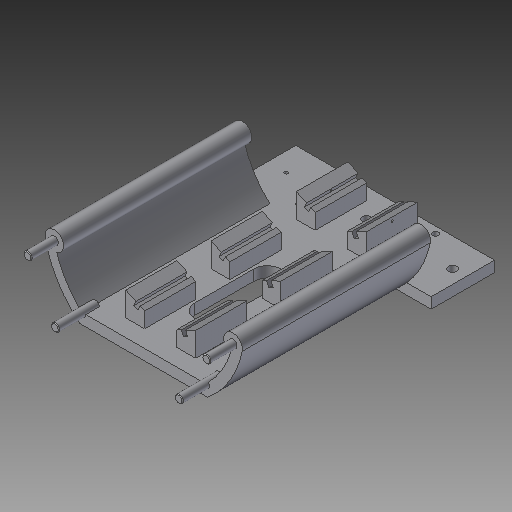
# Autodesk Inventor part: 3214_Bed Rail End_V1
Saved by Autodesk Inventor 2020 (Build 240168000, 168)
## iProperties
Created: 2019-06-18
Part Number: 3214_Bed Rail End_V1
Material: Acetal Resin, White
Document SubType Name: Sheet Metal
Designer: MPI
Density: 1.425 g/cm^3
Sheet Metal Rule: Default_mm
Appearance: Smooth - White
Mass: 455.781 g
Surface Area: 903.238 cm^2
Volume: 319.846 cm^3
Author: MPI
Autodesk Inventor part; units mm, degrees
ref_plane "YZ Plane" through (0, 0, 0) normal (1, 0, 0) x (0, 1, 0)
sketch "Sketch19" plane through (0, 0, 0) normal (0, 0, 1) x (1, 0, 0)
  line L0 (47.55, -58) -> (-47.55, -58)
  line L1 (-100, -14) -> (156, -14) construction
  arc A0 (47.55, -58) -> (73.6817, -14) centre (0, 0) ccw
  arc A1 (-73.6817, -14) -> (-47.55, -58) centre (0, 0) ccw
  arc A2 (-64.7514, -20.7668) -> (-73.3933, -15.4412) centre (-66.5432, -14) ccw
  arc A3 (73.3933, -15.4412) -> (64.7514, -20.7668) centre (66.5432, -14) ccw
  arc A4 (-67.6299, -7.0849) -> (-64.8992, -20.3) centre (0, 0) ccw construction
  arc A5 (-64.7514, -20.7668) -> (-46.0869, -50) centre (0, 0) ccw
  arc A6 (46.0869, -50) -> (64.7514, -20.7668) centre (0, 0) ccw
  arc A7 (64.8058, -20.5962) -> (67.6299, -7.0849) centre (0, 0) ccw construction
  line L2 (0, 0) -> (-33.9351, 15.8242) construction
  line L3 (0, 0) -> (37.291, 17.3891) construction
  line L4 (0, 0) -> (0, -41) construction
  line L5 (0, 0) -> (-21.2237, -45.5143) construction
  line L6 (0, 0) -> (17.7082, -37.9755) construction
  line L7 (-12, -38.5394) -> (-12, -50)
  line L8 (12, -38.5394) -> (12, -50)
  line L9 (-26, -32.0111) -> (-26, -50)
  line L10 (26, -32.0111) -> (26, -50)
  line L11 (-18.4455, -35.5339) -> (-20.1359, -39.1591)
  line L12 (-20.1359, -39.1591) -> (-17.0545, -40.596)
  line L13 (-17.0545, -40.596) -> (-15.364, -36.9708)
  line L14 (15.364, -36.9708) -> (17.0545, -40.596)
  line L15 (17.0545, -40.596) -> (20.1359, -39.1591)
  line L16 (20.1359, -39.1591) -> (18.4455, -35.5339)
  line L17 (-12, -38.5394) -> (-15.364, -36.9708)
  line L18 (-18.4455, -35.5339) -> (-26, -32.0111)
  line L19 (12, -38.5394) -> (15.364, -36.9708)
  line L20 (18.4455, -35.5339) -> (26, -32.0111)
  line L21 (-46.0869, -50) -> (-26, -50)
  line L22 (-12, -50) -> (12, -50)
  line L23 (26, -50) -> (46.0869, -50)
  dimension "d378" = 58
  dimension "d379" = 14
  dimension "d381" = 75
  dimension "d383" = 75
  dimension "d384" = 14
  dimension "d385" = 14
  dimension "d389" = 25
  dimension "d390" = 25
  dimension "d391" = 90
  dimension "d392" = 90
  dimension "d393" = 24
  dimension "d394" = 12
  dimension "d395" = 14
  dimension "d396" = 14
  dimension "d399" = 3.4
  dimension "d400" = 4
  dimension "d401" = 1.7
  dimension "d402" = 3.4
  dimension "d403" = 1.7
  dimension "d404" = 4
  constraints: 48 end point, 20 point on circle, 11 perpendicular, 8 centre point, 8 parallel, 4 horizontal, 2 coincident, 2 point on line, 2 vertical
  measures "d378" distance from line of L0 point (0, 0)
  measures "d379" distance from line of L1 point (0, 0)
  measures "d381" radius of A1
  measures "d383" radius of A0
  measures "d384" diameter of A2
  measures "d385" diameter of A3
  measures "d389" angle of L4 L6
  measures "d390" angle of L4 L5
  measures "d391" angle of L5 L2
  measures "d392" angle of L6 L3
  measures "d393" distance between parallel lines of L8 L7
  measures "d394" distance between parallel lines of L4 L7
  measures "d395" distance between parallel lines of L7 L9
  measures "d396" distance between parallel lines of L10 L8
  measures "d399" distance between parallel lines of L13 L11
  measures "d400" distance of L12.end L13.end
  measures "d401" distance between parallel lines of L5 L13
  measures "d402" distance between parallel lines of L16 L14
  measures "d403" distance between parallel lines of L6 L14
  measures "d404" distance of L14.start L14.end
extrude "Extrusion17" add sketch "Sketch19" along normal blind 140
sketch "Sketch20" plane through (0, 0, 0) normal (0, 0, -1) x (-1, 0, 0)
  line L0 (74, -50) -> (74, -58)
  line L1 (74, -58) -> (-74, -58)
  line L2 (-74, -58) -> (-74, -50)
  line L3 (47.55, -58) -> (-47.55, -58) projected
  line L4 (26, -50) -> (46.0869, -50) projected
  line L5 (-46.0869, -50) -> (-26, -50) projected
  line L6 (-26, -50) -> (-26, -32.0111)
  line L7 (-26, -32.0111) -> (-18.4455, -35.5339)
  line L8 (-18.4455, -35.5339) -> (-20.1359, -39.1591)
  line L9 (-20.1359, -39.1591) -> (-17.0545, -40.596)
  line L10 (-17.0545, -40.596) -> (-15.364, -36.9708)
  line L11 (-15.364, -36.9708) -> (-12, -38.5394)
  line L12 (-12, -38.5394) -> (-12, -50)
  line L13 (-12, -50) -> (12, -50) projected
  line L14 (12, -50) -> (12, -38.5394)
  line L15 (12, -38.5394) -> (15.364, -36.9708)
  line L16 (17.0545, -40.596) -> (20.1359, -39.1591)
  line L17 (20.1359, -39.1591) -> (18.4455, -35.5339)
  line L18 (18.4455, -35.5339) -> (26, -32.0111)
  line L19 (26, -32.0111) -> (26, -50)
  line L20 (26, -32.0111) -> (26, -50) projected
  line L21 (20.1359, -39.1591) -> (18.4455, -35.5339) projected
  line L22 (12, -50) -> (12, -38.5394) projected
  line L23 (12, -38.5394) -> (15.364, -36.9708) projected
  line L24 (15.364, -36.9708) -> (17.0545, -40.596)
  line L25 (15.364, -36.9708) -> (17.0545, -40.596) projected
  line L26 (-26, -50) -> (-26, -32.0111) projected
  line L27 (-12, -38.5394) -> (-12, -50) projected
  line L28 (-20.1359, -39.1591) -> (-17.0545, -40.596) projected
  line L29 (-17.0545, -40.596) -> (-15.364, -36.9708) projected
  line L30 (-15.364, -36.9708) -> (-12, -38.5394) projected
  line L31 (-26, -32.0111) -> (-18.4455, -35.5339) projected
  line L32 (-18.4455, -35.5339) -> (-20.1359, -39.1591) projected
  line L33 (-74, -50) -> (-26, -50)
  line L34 (-12, -50) -> (12, -50)
  line L35 (26, -50) -> (74, -50)
  point P0 (0, 0)
  dimension "d407" = 148
  dimension "d408" = 74
  constraints: 44 end point, 16 collinear, 8 perpendicular, 5 parallel, 3 horizontal, 3 point on line, 2 vertical
  measures "d407" distance between parallel lines of L0 L2
  measures "d408" distance from line of point (0, 0) L2
extrude "Extrusion18" add sketch "Sketch20" along normal blind 38.1
sketch "Sketch21" plane through (-12, -50, 140) normal (0, 1, 0) x (1, 0, 0)
  line L0 (48, 0) -> (-24, 0)
  line L1 (-24, 0) -> (-24, 12.7)
  line L2 (-24, 12.7) -> (48, 12.7)
  line L3 (48, 12.7) -> (48, 0)
  line L4 (48, 50.8) -> (-24, 50.8)
  line L5 (-24, 50.8) -> (-24, 76.2)
  line L6 (-24, 76.2) -> (48, 76.2)
  line L7 (48, 76.2) -> (48, 50.8)
  line L8 (48, 114.3) -> (-24, 114.3)
  line L9 (-24, 114.3) -> (-24, 139.7)
  line L10 (-24, 139.7) -> (48, 139.7)
  line L11 (48, 139.7) -> (48, 114.3)
  line L12 (24, 0) -> (0, 0) projected
  line L13 (38, 178.1) -> (38, 0) projected
  line L14 (-14, 178.1) -> (-14, 0) projected
  point P0 (12, 140)
  dimension "d412" = 10
  dimension "d413" = 10
  dimension "d414" = 12.7
  dimension "d415" = 38.1
  dimension "d416" = 25.4
  dimension "d417" = 38.1
  dimension "d418" = 25.4
  constraints: 24 end point, 6 parallel, 3 horizontal, 3 perpendicular, 3 point on line, 2 collinear
  measures "d412" distance between parallel lines of L13 L3
  measures "d413" distance between parallel lines of L14 L1
  measures "d414" distance of L0.end L1.end
  measures "d415" distance between parallel lines of L4 L2
  measures "d416" distance between parallel lines of L6 L4
  measures "d417" distance between parallel lines of L8 L6
  measures "d418" distance between parallel lines of L8 L10
extrude "Extrusion19" cut sketch "Sketch21" along normal up to next contours L0 L13 L2 L3 | L0 L14 L2 L13 | L14 L0 L1 L2 | L13 L6 L7 L4 | L4 L14 L6 L13 | L4 L5 L6 L14 | L13 L10 L11 L8 | L8 L14 L10 L13 | L8 L9 L10 L14
sketch "Sketch22" plane through (0, 0, 140) normal (0, 0, 1) x (1, 0, 0)
  arc A0 (-64.7514, -20.7668) -> (-73.3933, -15.4412) centre (-66.5432, -14) ccw projected
  circle A1 centre (-66.5432, -14) radius 3
  arc A2 (73.3933, -15.4412) -> (64.7514, -20.7668) centre (66.5432, -14) ccw projected
  circle A3 centre (66.5432, -14) radius 3
  arc A4 (-64.7514, -20.7668) -> (-46.0869, -50) centre (0, 0) ccw projected
  circle A5 centre (-46.0869, -50) radius 3
  arc A6 (46.0869, -50) -> (64.7514, -20.7668) centre (0, 0) ccw projected
  circle A7 centre (46.0869, -50) radius 3
  dimension "d421" = 6
  dimension "d422" = 6
  dimension "d423" = 6
  dimension "d424" = 6
  constraints: 4 centre point, 2 coincident, 2 other
  measures "d421" diameter of A1
  measures "d422" diameter of A3
  measures "d423" diameter of A5
  measures "d424" diameter of A7
extrude "Extrusion20" add sketch "Sketch22" along normal blind 20 and the other way blind 10
fillet "Fillet1" radius 0.5 4 edges at (-69.5432, -14, 160) (-49.0869, -50, 160) (43.0869, -50, 160) (63.5432, -14, 160)
sketch "Sketch23" plane through (55.9017, -50, 0) normal (0, 1, 0) x (1, 0, 0)
  circle A0 centre (-115.9017, 26.1) radius 1.3
  line L0 (-129.9017, 0) -> (-129.9017, 38.1) projected
  line L1 (18.0983, 0) -> (18.0983, 38.1) projected
  line L2 (-129.9017, 38.1) -> (-81.9017, 38.1) projected
  line L3 (-29.9017, 38.1) -> (18.0983, 38.1) projected
  circle A1 centre (-55.9017, 26.1) radius 3.25
  line L4 (-67.9017, 38.1) -> (-43.9017, 38.1) projected
  circle A2 centre (8.0983, 26.1) radius 3.25
  point P0 (-55.9017, 0)
  dimension "d430" = 2.6
  dimension "d431" = 14
  dimension "d433" = 12
  dimension "d435" = 6.5
  dimension "d436" = 0
  dimension "d437" = 12
  dimension "d453" = 6.5
  dimension "d454" = 12
  dimension "d455" = 10
  constraints: 3 centre point
  measures "d430" diameter of A0
  measures "d431" distance from line of A0.centre L0
  measures "d433" distance from line of L2 A0.centre
  measures "d435" diameter of A1
  measures "d436" horizontal distance of A1.centre point (-55.902, 0)
  measures "d437" distance from line of L4 A1.centre
  measures "d453" diameter of A2
  measures "d454" distance from line of L3 A2.centre
  measures "d455" distance from line of L1 A2.centre
extrude "Extrusion21" cut sketch "Sketch23" against normal through all
ref_plane "Work Plane3" through (-28.9586, -30.6315, -38.1) normal (-0.9063, 0.4226, 0) x (0, 0, 1)
sketch "Sketch24" plane through (-28.9586, -30.6315, -38.1) normal (-0.9063, 0.4226, 0) x (0, 0, 1)
  circle A0 centre (19.05, -2.5) radius 0.75
  line L0 (0, 0) -> (38.4, 0) projected
  line L1 (0, -16.3035) -> (0, 0) projected
  point P0 (38.1, 40)
  dimension "d441" = 1.5
  dimension "d442" = 2.5
  dimension "d443" = 19.05
  constraints: 1 centre point
  measures "d441" diameter of A0
  measures "d442" distance from line of A0.centre L0
  measures "d443" distance from line of A0.centre L1
extrude "Extrusion22" cut sketch "Sketch24" against normal blind 12
ref_plane "Work Plane4" through (30.6491, -34.2567, 0.3) normal (0.9063, 0.4226, 0) x (0, 0, -1)
sketch "Sketch25" plane through (30.6491, -34.2567, 0.3) normal (0.9063, 0.4226, 0) x (0, 0, -1)
  circle A0 centre (19.35, 1.5) radius 0.75
  line L0 (38.4, 4) -> (38.4, -12.3035) projected
  line L1 (38.4, 4) -> (0, 4) projected
  point P0 (0.3, 44)
  dimension "d447" = 19.05
  dimension "d448" = 1.5
  dimension "d450" = 2.5
  constraints: 1 centre point
  measures "d447" distance from line of L0 A0.centre
  measures "d448" diameter of A0
  measures "d450" distance from line of L1 A0.centre
extrude "Extrusion23" cut sketch "Sketch25" against normal blind 12
sketch "Sketch26" plane through (55.9017, -50, 0) normal (0, 1, 0) x (1, 0, 0)
  line L0 (-45.9017, -92) -> (-45.9017, -48)
  line L1 (-65.9017, -48) -> (-65.9017, -92)
  arc A0 (-65.9017, -92) -> (-45.9017, -92) centre (-55.9017, -92) ccw
  arc A1 (-45.9017, -48) -> (-65.9017, -48) centre (-55.9017, -48) ccw
  line L2 (-12.8148, -140) -> (-98.9886, -140) projected
  point P0 (-55.9017, 0)
  dimension "d456" = 20
  dimension "d457" = 10
  dimension "d458" = 44
  constraints: 4 end point, 4 point on circle, 2 centre point, 1 parallel
  measures "d456" distance of L0.end L1.start
  measures "d457" distance from line of point (-55.902, 0) L0
  measures "d458" distance of L0.start L0.end
extrude "Extrusion24" cut sketch "Sketch26" against normal through all
sketch "Sketch27" plane through (0, 0, -38.1) normal (0, 0, -1) x (-1, 0, 0)
  line L0 (-74, -50) -> (-74, -58) projected
  line L1 (-74, -58) -> (74, -58) projected
  line L2 (74, -58) -> (74, -50) projected
  line L3 (74, -50) -> (26, -50) projected
  line L4 (26, -50) -> (26, -32.0111) projected
  line L5 (26, -32.0111) -> (18.4455, -35.5339) projected
  line L6 (18.4455, -35.5339) -> (20.1359, -39.1591) projected
  line L7 (20.1359, -39.1591) -> (17.0545, -40.596) projected
  line L8 (17.0545, -40.596) -> (15.364, -36.9708) projected
  line L9 (15.364, -36.9708) -> (12, -38.5394) projected
  line L10 (12, -38.5394) -> (12, -50) projected
  line L11 (12, -50) -> (-12, -50) projected
  line L12 (-12, -50) -> (-12, -38.5394) projected
  line L13 (-12, -38.5394) -> (-15.364, -36.9708) projected
  line L14 (-15.364, -36.9708) -> (-17.0545, -40.596) projected
  line L15 (-17.0545, -40.596) -> (-20.1359, -39.1591) projected
  line L16 (-20.1359, -39.1591) -> (-18.4455, -35.5339) projected
  line L17 (-18.4455, -35.5339) -> (-26, -32.0111) projected
  line L18 (-26, -32.0111) -> (-26, -50) projected
  line L19 (-26, -50) -> (-74, -50) projected
  line L20 (-74, -50) -> (-74, -58) projected
  line L21 (74, -50) -> (55.9017, -50) projected
  line L22 (-74, -58) -> (74, -58)
  line L23 (74, -58) -> (74, -50)
  line L24 (74, -50) -> (-74, -50)
  line L25 (-74, -50) -> (-74, -58)
  point P0 (0, 0)
  constraints: 8 end point, 2 parallel, 1 horizontal, 1 perpendicular
extrude "Extrusion25" add sketch "Sketch27" along normal blind 9.15 contours L19 L24 L11 L3 L2 L1 L0
sketch "Sketch28" plane through (-74, -50, 0) normal (0, 1, 0) x (1, 0, 0)
  line L0 (109, 42.25) -> (39, 42.25) construction
  line L1 (39, 42.25) -> (39, 11.25) construction
  line L2 (39, 11.25) -> (109, 11.25) construction
  line L3 (109, 11.25) -> (109, 42.25) construction
  line L4 (0, 47.25) -> (148, 47.25) construction
  point P0 (74, 0)
  point P1 (74, 42.25)
  point P2 (74, 47.25)
  dimension "d464" = 70
  dimension "d465" = 31
  dimension "d466" = 5
  constraints: 8 end point, 4 coincident, 2 midpoint, 2 parallel, 1 horizontal, 1 perpendicular, 1 vertical alignment
  measures "d464" distance of L0.start L0.end
  measures "d465" distance of L2.end L0.start
  measures "d466" distance between parallel lines of L4 L0
hole "Hole1" at (35, -50, -11.25) at (35, -50, -42.25) at (-35, -50, -42.25) at (-35, -50, -11.25) direction (0, -1, 0) diameter 4.5 end through all clearance for "Flat Head Machine Screw" size "M4" standard "Ansi Metric M Profile"
equation "\"BendRadius\" = Thickness"
equation "\"BendReliefWidth\" = Thickness"
equation "\"BendReliefDepth\" = 0.5 * Thickness"
equation "\"CornerReliefSize\" = 4 * Thickness"
equation "\"MinimumRemnant\" = 2 * Thickness"
equation "\"TransitionRadius\" = BendRadius"
equation "\"JacobiRadiusSize\" = BendRadius"
equation "\"GapSize\" = Thickness"
equation "\"Thickness\" = 0.5"
body "Solid2"
